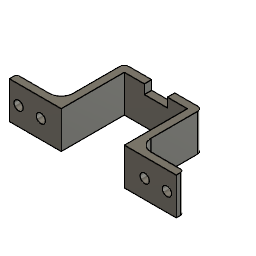
krep_motora (Autodesk Fusion 360 design; units mm, degrees)
Autodesk Fusion 360 part; units mm, degrees
sketch "Sketch1" plane through (0, 0, 0) normal (0, 1, 0) x (1, 0, 0)
  line L0 (21.25, -21.25) -> (-21.25, -21.25)
  line L1 (-21.25, -21.25) -> (-21.25, 21.25)
  line L2 (-21.25, 21.25) -> (21.25, 21.25)
  line L3 (21.25, 21.25) -> (21.25, -21.25)
  line L4 (21.25, -21.25) -> (-21.25, 21.25) construction
  line L5 (-21.25, -21.25) -> (21.25, 21.25) construction
  line L6 (-21.25, -21.25) -> (-56.25, -21.25)
  line L7 (-56.25, -21.25) -> (-56.25, -16.25)
  line L8 (-56.25, -16.25) -> (-21.25, -16.25)
  line L9 (0, -21.25) -> (0, -35)
  line L10 (-26.25, -21.25) -> (-26.25, 26.25)
  line L11 (-26.25, 26.25) -> (26.25, 26.25)
  line L12 (26.25, 26.25) -> (26.25, -21.25)
  line L13 (56.25, -16.25) -> (21.25, -16.25)
  line L14 (21.25, -21.25) -> (56.25, -21.25)
  line L15 (56.25, -21.25) -> (56.25, -16.25)
  dimension "d1" = 42.5
  dimension "d2" = 42.5
  dimension "d3" = 35
  dimension "d4" = 5
  constraint horizontal L0
  constraint perpendicular L0 L1
  constraint parallel L0 L2
  constraint parallel L1 L3
  constraint coincident L4 origin
  constraint coincident L5 origin
  constraint perpendicular L1 L6
  constraint perpendicular L6 L7
  constraint coincident L1 L8.end
  constraint perpendicular L1 L8
  constraint midpoint L0 L9.start
  constraint perpendicular L0 L9
  constraint coincident L6 L10.start
  constraint symmetric L0.end L9 L0.start
  constraint symmetric L6.end L9 L14.end
  constraint symmetric L7.end L9 L13.start
  constraint symmetric L8.end L9 L13.end
  constraint coincident L14 L12.end
  measures "d1" distance of L1.end L2.end
  measures "d2" distance of L0.end L1.end
  measures "d3" distance of L0.end L6.end
  measures "d4" distance of L6.end L7.end
extrude "Extrude1" add sketch "Sketch1" along normal blind 25 contours L3 L12 L13 L14 | L1 L2 L3 L8 L10 L11 L12 L13 | L12 L13 L14 L15 | L1 L6 L8 L10 | L6 L7 L8 L10
sketch "Sketch2" plane through (0, 0, 16.25) normal (0, 0, -1) x (-1, 0, 0)
  line L0 (26.25, 0) -> (56.25, 0)
  line L1 (56.25, 0) -> (56.25, 25)
  line L2 (56.25, 25) -> (26.25, 25)
  line L3 (26.25, 25) -> (26.25, 0)
  line L4 (0, 12.5) -> (0, 7)
  circle A0 centre (50, 12.5) radius 3.1
  circle A1 centre (35, 12.5) radius 3.1
  circle A2 centre (-35, 12.5) radius 3.1
  circle A3 centre (-50, 12.5) radius 3.1
  line L5 (0, 25) -> (7.75, 25)
  line L6 (0, 18.75) -> (7.75, 18.75)
  line L7 (7.75, 18.75) -> (7.75, 25)
  line L8 (0, 18.75) -> (-7.75, 18.75)
  line L9 (-7.75, 18.75) -> (-7.75, 25)
  line L10 (0, 25) -> (-7.75, 25)
  point P0 (0, 12.5)
  dimension "d8" = 6.2
  dimension "d9" = 6.2
  dimension "d10" = 7.75
  constraint symmetric L4 A0 A3
  constraint symmetric L4 A1 A2
  constraint horizontal L5
  constraint coincident P0 L4.start
  constraint perpendicular L5 L7
  measures "d8" diameter of A0
  measures "d9" diameter of A1
  measures "d10" distance of L5.start L5.end
extrude "Extrude2" cut sketch "Sketch2" along normal mid plane 144 contours A0 | A1 | A2 | A3 | L5 L6 L7 L8 L9 L10
fillet "Fillet1" radius 8 2 edges at (-26.25, 12.5, 16.25) (26.25, 12.5, 16.25)
fillet "Fillet2" radius 3 2 edges at (-26.25, 12.5, -26.25) (26.25, 12.5, -26.25)
fillet "Fillet3" radius 2 2 edges at (-56.25, 12.5, 16.25) (56.25, 12.5, 16.25)
